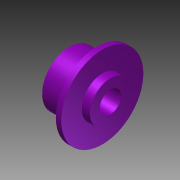
# Autodesk Inventor part: SensorSkiva Plugg
Saved by Autodesk Inventor 2012 SP1 (Build 160190100, 190)
## iProperties
Created: 2014-02-18
Part Number: SensorSkiva Plugg
Material: Default
Document SubType Name: Modeling
Designer: Pinkponk
Density: 1 g/cm^3
Author: Pinkponk
Autodesk Inventor part; units mm, degrees
ref_plane "YZ Plane" through (0, 0, 0) normal (1, 0, 0) x (0, 1, 0)
ref_plane "XZ Plane" through (0, 0, 0) normal (0, 1, 0) x (-1, 0, 0)
ref_plane "XY Plane" through (0, 0, 0) normal (0, 0, 1) x (1, 0, 0)
sketch "Sketch1" plane through (0, 0, 0) normal (0, 0, 1) x (1, 0, 0)
  line L0 (0, 10) -> (10, 10)
  line L1 (10, 10) -> (10, 15)
  line L2 (10, 15) -> (12, 15)
  line L3 (12, 15) -> (12, 7.5)
  line L4 (12, 7.5) -> (15, 7.5)
  line L5 (0, 0) -> (21.5925, 0)
  line L6 (0, 10) -> (0, 3.9)
  line L7 (0, 3.9) -> (15, 3.9)
  line L8 (15, 7.5) -> (15, 3.9)
  point P0 (12, 11.25)
  dimension "d0" = 20
  dimension "d1" = 7.8
  dimension "d3" = 30
  dimension "d4" = 15
  dimension "d6" = 10
  dimension "d7" = 2
  dimension "d10" = 3
  constraints: 18 end point, 3 perpendicular, 2 parallel, 2 vertical alignment, 1 horizontal, 1 midpoint, 1 vertical
  measures "d0" diameter of L0 L5
  measures "d1" diameter of L7 L5
  measures "d3" diameter of L2 L5
  measures "d4" diameter of L4 L5
  measures "d6" distance of L0.start L0.end
  measures "d7" distance of L1.end L2.end
  measures "d10" distance of L3.end L4.end
revolve "Revolution1" add sketch "Sketch1" angle 360 about axis through (0, 0, 0) along (1, 0, 0)
body "Solid1"
